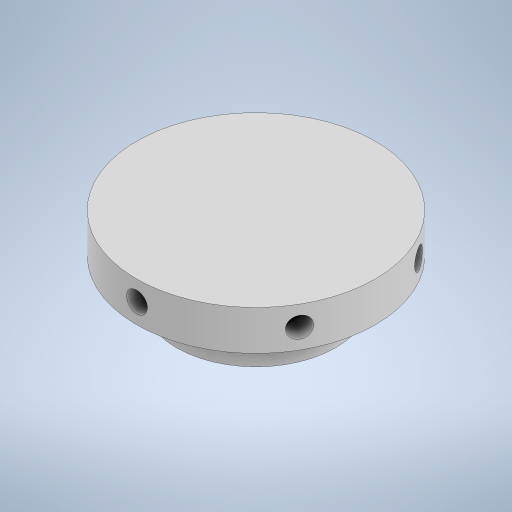
# Autodesk Inventor part: exp_tire_6rod_rev0
Saved by Autodesk Inventor 2024 (Build 280153000, 153)
## iProperties
Created: 2024-04-09
Part Number: exp_tire_6rod_rev0
Material: 一般
Document SubType Name: Modeling
Designer: Akio
Density: 1 g/cm^3
Appearance: 既定
Author: Akio
Autodesk Inventor part; units mm, degrees
ref_plane "YZ Plane" through (0, 0, 0) normal (1, 0, 0) x (0, 1, 0)
ref_plane "XZ Plane" through (0, 0, 0) normal (0, 1, 0) x (-1, 0, 0)
sketch "スケッチ1" plane through (0, 0, 0) normal (0, 1, 0) x (-1, 0, 0)
  circle A0 centre (0, 0) radius 10
  dimension "d0" = 20
  constraints: 1 centre point, 1 coincident
  measures "d0" diameter of A0
extrude "押し出し1" add sketch "スケッチ1" along normal blind 5
sketch "スケッチ2" plane through (0, 5, 0) normal (0, 1, 0) x (1, 0, 0)
  circle A0 centre (0, 0) radius 15
  dimension "d3" = 30
  constraints: 1 centre point, 1 coincident
  measures "d3" diameter of A0
extrude "押し出し2" add sketch "スケッチ2" along normal blind 5
sketch "スケッチ5" plane through (0, 0, 0) normal (0, -1, 0) x (1, 0, 0)
  line L0 (0, 1.5588) -> (1.35, 0.7794)
  line L1 (1.35, 0.7794) -> (1.35, -0.7794)
  line L2 (1.35, -0.7794) -> (0, -1.5588)
  line L3 (0, -1.5588) -> (-1.35, -0.7794)
  line L4 (-1.35, -0.7794) -> (-1.35, 0.7794)
  line L5 (-1.35, 0.7794) -> (0, 1.5588)
  point P0 (0, 0)
  point P1 (0, 0)
  dimension "d14" = 2.7
  constraints: 12 end point, 1 coincident, 13 other
  measures "d14" distance between parallel lines of L1 L4
extrude "押し出し3" cut sketch "スケッチ5" against normal blind 5
ref_plane "作業平面1" through (0, 0, 3) normal (0, 0, 1) x (1, 0, 0)
sketch "スケッチ8" plane through (0, 0, 3) normal (0, 0, 1) x (1, 0, 0)
  circle A0 centre (0, 7.5) radius 1.3
  line L0 (15, 10) -> (-15, 10) projected
  point P0 (0, 0)
  dimension "d22" = 2.6
  dimension "d23" = 2.5
  constraints: 1 centre point
  measures "d22" diameter of A0
  measures "d23" distance from line of L0 A0.centre
extrude "押し出し5" cut sketch "スケッチ8" along normal through all
pattern_circular "円形状パターン1" count 6 over 360 about axis through (0, 5, 0) along (0, 1, 0) of "押し出し5"
